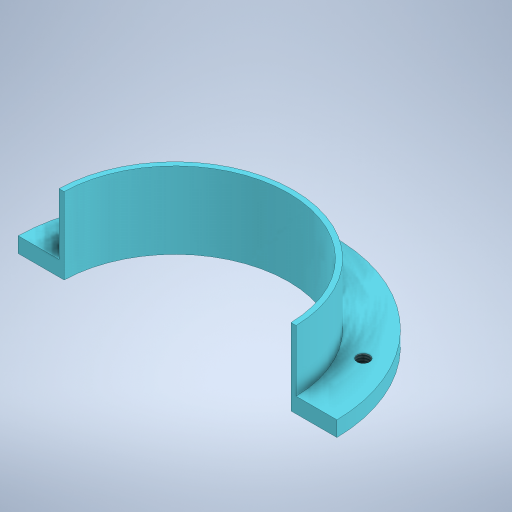
# Autodesk Inventor part: LowerClamp
Saved by Autodesk Inventor 2024 (Build 280153000, 153)
## iProperties
Created: 2023-10-26
Part Number: LowerClamp
Material: Brass, Soft Yellow
Document SubType Name: Modeling
Designer: schanen
Density: 8.47 g/cm^3
Appearance: Cadet Blue
Author: schanen
Autodesk Inventor part; units mm, degrees
ref_plane "YZ Plane" through (0, 0, 0) normal (1, 0, 0) x (0, 1, 0)
ref_plane "XZ Plane" through (0, 0, 0) normal (0, 1, 0) x (-1, 0, 0)
ref_plane "XY Plane" through (0, 0, 0) normal (0, 0, 1) x (1, 0, 0)
sketch "Sketch1" plane through (0, 0, 0) normal (0, 0, 1) x (1, 0, 0)
  line L0 (-31.225, 0) -> (-22.225, 0)
  line L1 (-22.225, 0) -> (-22.225, 15)
  line L2 (-22.225, 15) -> (-23.225, 15)
  line L3 (-23.225, 15) -> (-23.225, 3)
  line L4 (-23.225, 3) -> (-31.225, 3)
  line L5 (-31.225, 3) -> (-31.225, 0)
  line L6 (0, -3) -> (0, 18) projected
  point P0 (0, 0)
  dimension "d0" = 3
  dimension "d1" = 1
  dimension "d2" = 15
  dimension "d3" = 22.225
  dimension "d17" = 9
  constraints: 12 end point, 4 perpendicular, 1 horizontal, 1 horizontal alignment, 1 parallel
  measures "d0" distance of L4.end L0.start
  measures "d1" distance between parallel lines of L1 L3
  measures "d2" distance of L0.end L1.end
  measures "d3" distance from line of point (0, 0) L1
  measures "d17" distance of L0.start L0.end
revolve "Revolution1" add sketch "Sketch1" angle 360 about axis through (0, -10, 0) along (0, 1, 0)
sketch "Sketch2" plane through (0, 3, 0) normal (0, 1, 0) x (1, 0, 0)
  point P0 (0, 0)
  point P1 (0, 27)
  dimension "d6" = 27
  constraints: 1 vertical alignment
  measures "d6" distance of point (0, 0) point (0, 27)
hole "Hole1" at (0, 3, -27) direction (0, -1, 0) diameter 2.459 end through all thread size "M3x0.5" class "6H" standard "ISO Metric profile"
sketch "Sketch3" plane through (0, 15, 0) normal (0, 1, 0) x (1, 0, 0)
  line L0 (-31.225, 0.5) -> (31.225, 0.5)
  line L1 (31.225, 0.5) -> (31.225, -31.225)
  line L2 (31.225, -31.225) -> (-31.225, -31.225)
  line L3 (-31.225, -31.225) -> (-31.225, 0.5)
  circle A0 centre (0, 0) radius 31.225 projected
  circle A1 centre (0, 0) radius 23.225 projected
  point P0 (31.225, 0)
  point P1 (31.221, 0.5)
  point P2 (-31.221, 0.5)
  point P3 (-31.225, 0)
  point P4 (0, -31.225)
  point P5 (23.2196, 0.5)
  point P6 (-23.2196, 0.5)
  dimension "d14" = 0.5
  constraints: 8 end point, 3 tangent, 2 parallel, 1 horizontal, 1 perpendicular
  measures "d14" distance from line of point (0, 0) L0
extrude "Extrusion1" cut sketch "Sketch3" against normal blind 15 contours L0 A1 A0 | A0 L2 L3 | L0 A1 | A0 L1 L2 picked at (-27.077, -8.535) picked at (5.7691, -4.8291)
pattern_circular "Circular Pattern1" count 6 over 360 about axis through (0, 7.5, 0) along (0, 1, 0) of "Hole1"
body "Solid1"
